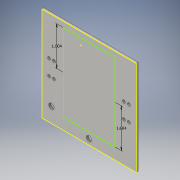
# Autodesk Inventor part: mcdave_FRAME
Saved by Autodesk Inventor 2016 (Build 200138000, 138)
## iProperties
Created: 2017-09-08
Part Number: mcdave_FRAME
Material: Generic
Document SubType Name: Modeling
Designer: student
Density: 1 g/cm^3
Appearance: Default
Author: student
Autodesk Inventor part; units mm, degrees
ref_plane "YZ Plane" through (0, 0, 0) normal (1, 0, 0) x (0, 1, 0)
ref_plane "XZ Plane" through (0, 0, 0) normal (0, 1, 0) x (-1, 0, 0)
ref_plane "XY Plane" through (0, 0, 0) normal (0, 0, 1) x (1, 0, 0)
sketch "Sketch1" plane through (0, 0, 0) normal (0, 0, 1) x (1, 0, 0)
  line L0 (-41.0863, 12.6642) -> (57.9737, 12.6642)
  line L1 (57.9737, 12.6642) -> (57.9737, -86.3958)
  line L2 (57.9737, -86.3958) -> (-41.0863, -86.3958)
  line L3 (-41.0863, -86.3958) -> (-41.0863, 12.6642)
  point P0 (0, 0)
  dimension "d0" = 99.06
  dimension "d1" = 99.06
  constraints: 8 end point, 2 parallel, 1 horizontal, 1 perpendicular
  measures "d0" distance of L0.start L0.end
  measures "d1" distance of L0.end L1.end
extrude "Extrusion1" add sketch "Sketch1" along normal blind 2.032
sketch "Sketch5" plane through (0, 0, 2.032) normal (0, 0, 1) x (1, 0, 0)
  line L0 (-41.0863, 12.6642) -> (-41.0863, -86.3958) projected
  line L1 (57.9737, -86.3958) -> (57.9737, 12.6642) projected
  line L2 (57.9737, 12.6642) -> (-41.0863, 12.6642) projected
  line L3 (35.4947, -33.7662) -> (35.4947, -74.4951)
  line L4 (35.4947, -74.4951) -> (-18.6073, -74.4951)
  line L5 (-18.6073, -74.4951) -> (-18.6073, -33.7662)
  line L6 (-18.6073, -33.7662) -> (-18.6073, 6.9627)
  line L7 (-18.6073, -74.4951) -> (-18.6073, 6.9627)
  line L8 (-18.6073, -74.4951) -> (35.4947, -74.4951)
  line L9 (-18.6073, 6.9627) -> (35.4947, 6.9627)
  line L10 (35.4947, 6.9627) -> (35.4947, -33.7662)
  line L11 (-41.0863, -86.3958) -> (57.9737, -86.3958) projected
  point P0 (0, 0)
  dimension "d14" = 40.7289
  dimension "d15" = 40.7289
  constraints: 16 end point, 2 collinear, 1 horizontal, 1 perpendicular, 1 point on line
  measures "d14" distance of L3.start L3.end
  measures "d15" distance of L5.end L6.end
sketch "Sketch9" plane through (0, 0, 2.032) normal (0, 0, 1) x (1, 0, 0)
  line L0 (57.9737, -86.3958) -> (-41.0863, -86.3958) projected
  circle A0 centre (8.4437, -80.5421) radius 2.7051
  line L1 (-41.0863, -86.3958) -> (57.9737, -86.3958) projected
  point P0 (0, 0)
  dimension "d28" = 5.4102
  constraints: 1 centre point
  measures "d28" diameter of A0
extrude "Extrusion8" cut sketch "Sketch9" against normal through all
sketch "Sketch10" plane through (0, 0, 2.032) normal (0, 0, 1) x (1, 0, 0)
  circle A0 centre (-30.9416, -70.8163) radius 2.8321
  point P0 (0, 0)
  dimension "d31" = 5.6642
  constraints: 1 centre point
  measures "d31" diameter of A0
extrude "Extrusion9" cut sketch "Sketch10" against normal through all
sketch "Sketch16" plane through (0, 0, 2.032) normal (0, 0, 1) x (1, 0, 0)
  circle A0 centre (-33.4176, -44.7238) radius 1.5094
  circle A1 centre (-28.2679, -44.7238) radius 1.5113
  circle A2 centre (-28.2679, -44.7238) radius 1.5113
  circle A3 centre (-28.2999, -28.4285) radius 1.5113
  circle A4 centre (-33.4496, -28.4488) radius 1.5113
  circle A5 centre (-33.4496, -28.4488) radius 1.5113
  arc A6 (-36.3419, -47.086) -> (-35.8339, -47.594) centre (-35.8339, -47.086) ccw
  line L0 (57.9737, 12.6642) -> (-41.0863, 12.6642) projected
  line L1 (-41.0863, -86.3958) -> (57.9737, -86.3958) projected
  circle A7 centre (50.337, -28.4488) radius 1.5113
  circle A8 centre (50.337, -28.4488) radius 1.5113
  circle A9 centre (45.1874, -28.4285) radius 1.5113
  circle A10 centre (45.1554, -44.7238) radius 1.5113
  circle A11 centre (45.1554, -44.7238) radius 1.5113
  circle A12 centre (50.3051, -44.7238) radius 1.5094
  arc A13 (52.7213, -47.594) -> (53.2293, -47.086) centre (52.7213, -47.086) ccw
  point P0 (0, 0)
  point P1 (-36.3419, -26.0548)
  point P2 (-25.3437, -26.0548)
  point P3 (-25.3437, -47.086)
  point P4 (-25.8517, -47.594)
  point P5 (-28.2679, -44.7238)
  point P6 (53.2293, -26.0548)
  point P7 (42.2311, -26.0548)
  point P8 (42.2311, -47.086)
  point P9 (45.1554, -44.7238)
  point P10 (42.7391, -47.594)
  dimension "d50" = 3.0226
  constraints: 14 centre point, 6 coincident, 4 point on circle, 1 concentric
  measures "d50" diameter of A4
extrude "Extrusion11" cut sketch "Sketch16" against normal through all
body "Solid1"
